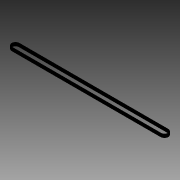
# Autodesk Inventor part: gt2Belt600
Saved by Autodesk Inventor 2013 (Build 170138000, 138)
## iProperties
Created: 2015-01-15
Part Number: gt2Belt600
Material: Generic
Document SubType Name: Modeling
Designer: dzban
Density: 1 g/cm^3
Author: dzban
Autodesk Inventor part; units mm, degrees
ref_plane "YZ Plane" through (0, 0, 0) normal (1, 0, 0) x (0, 1, 0)
ref_plane "XZ Plane" through (0, 0, 0) normal (0, 1, 0) x (-1, 0, 0)
ref_plane "XY Plane" through (0, 0, 0) normal (0, 0, 1) x (1, 0, 0)
sketch "Sketch1" plane through (0, 0, 0) normal (0, 0, 1) x (1, 0, 0)
  arc A0 (0, 6) -> (0, -6) centre (0, 0) ccw
  arc A1 (279, -6) -> (279, 6) centre (279, 0) ccw
  line L0 (0, -6) -> (279, -6)
  line L1 (279, 6) -> (0, 6)
  line L2 (0, 7.2) -> (279, 7.2)
  arc A2 (279, -7.2) -> (279, 7.2) centre (279, 0) ccw
  line L3 (279, -7.2) -> (0, -7.2)
  arc A3 (0, 7.2) -> (0, -7.2) centre (0, 0) ccw
  dimension "d0" = 12
  dimension "d2" = 12
  dimension "d3" = 279
  dimension "d4" = 1.2
  constraints: 8 end point, 8 point on circle, 4 centre point, 2 horizontal, 2 tangent, 1 coincident, 1 horizontal alignment, 3 other
  measures "d0" diameter of A0
  measures "d2" diameter of A1
  measures "d3" distance of A1.centre point (0, 0)
  measures "d4" distance between parallel lines of L0 L3
extrude "Extrusion1" add sketch "Sketch1" along normal blind 6
body "Solid1"
